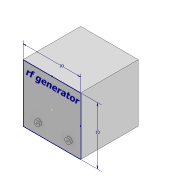
# Autodesk Inventor part: rf-generator
Saved by Autodesk Inventor 2021 (Build 250183000, 183)
## iProperties
Created: 2022-02-10
Part Number: rf-generator
Material: Типовые
Document SubType Name: Modeling
Designer: Тиннелла о Каллинике
Density: 1 g/cm^3
Appearance: По умолчанию
Author: Тиннелла о Каллинике
Autodesk Inventor part; units mm, degrees
ref_plane "YZ Plane" through (0, 0, 0) normal (1, 0, 0) x (0, 1, 0)
ref_plane "XZ Plane" through (0, 0, 0) normal (0, 1, 0) x (-1, 0, 0)
sketch "Эскиз1" plane through (0, 0, 0) normal (0, 0, 1) x (1, 0, 0)
  line L0 (-5, 5) -> (5, 5)
  line L1 (5, 5) -> (5, -5)
  line L2 (5, -5) -> (-5, -5)
  line L3 (-5, -5) -> (-5, 5)
  point P0 (0, 0)
  point P1 (0, 5)
  point P2 (5, 0)
  dimension "d0" = 10
  dimension "d1" = 10
  constraints: 8 end point, 2 midpoint, 2 parallel, 1 horizontal, 1 horizontal alignment, 1 perpendicular, 1 vertical alignment
  measures "d0" distance of L0.start L0.end
  measures "d1" distance of L0.end L1.end
extrude "Выдавливание1" add sketch "Эскиз1" against normal blind 10
sketch "Эскиз2" plane through (0, 0, 0) normal (0, 0, 1) x (1, 0, 0)
  line L0 (-4.6144, 4.1403) -> (8.1453, 4.1403) construction
  line L1 (8.1453, 4.1403) -> (8.1453, 2.1383) construction
  line L2 (8.1453, 2.1383) -> (-4.6144, 2.1383) construction
  line L3 (-4.6144, 2.1383) -> (-4.6144, 4.1403) construction
  point P0 (0, 0)
  constraints: 2 other
ref_plane "РабПлоскость1" through (0, 0, 0) normal (0, 0, 1) x (1, 0, 0)
sketch "Эскиз3" plane through (0, 0, 0) normal (0, 0, 1) x (1, 0, 0)
  circle A0 centre (-2.2997, -3.0689) radius 0.5
  circle A1 centre (3.0277, -3.0689) radius 0.5
  point P0 (0, 0)
  dimension "d5" = 1
  dimension "d6" = 1
  constraints: 2 centre point
  measures "d5" diameter of A0
  measures "d6" diameter of A1
extrude "Выдавливание2" add sketch "Эскиз3" along normal blind 0.3
sketch "Эскиз4" plane through (0, 0, 0) normal (0, 0, 1) x (1, 0, 0)
  circle A0 centre (-2.2997, -3.0689) radius 0.5 projected
  circle A1 centre (-2.2997, -3.0689) radius 0.1
  circle A2 centre (3.039, -3.0689) radius 0.1
  point P0 (0, 0)
  dimension "d9" = 0.2
  dimension "d10" = 0.2
  constraints: 2 centre point, 1 coincident
  measures "d9" diameter of A1
  measures "d10" diameter of A2
extrude "Выдавливание3" add sketch "Эскиз4" along normal blind 0.4 contours A1 | A2
